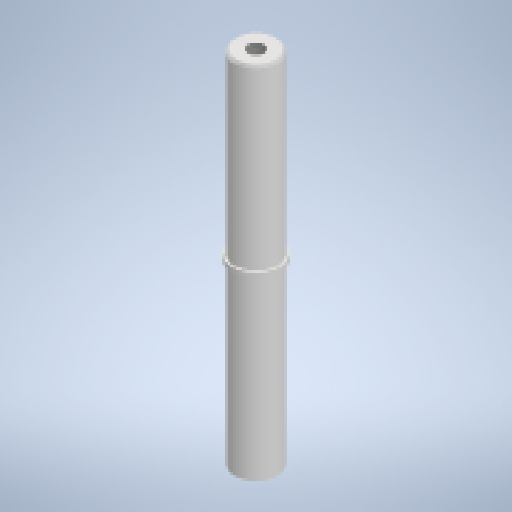
# Autodesk Inventor part: приводной вал
Saved by Autodesk Inventor 2024.2 (Build 282272000, 272)
## iProperties
Created: 2023-08-07
Part Number: приводной вал
Material: Generic
Document SubType Name: Modeling
Designer: admin
Density: 1 g/cm^3
Appearance: Default
Author: admin
Autodesk Inventor part; units mm, degrees
ref_plane "XZ Plane" through (0, 0, 0) normal (0, 1, 0) x (-1, 0, 0)
ref_plane "XY Plane" through (0, 0, 0) normal (0, 0, 1) x (1, 0, 0)
sketch "Sketch1" plane through (0, 0, 0) normal (0, 0, 1) x (1, 0, 0)
  line L0 (0, 75) -> (0, -75)
  line L1 (7, 75) -> (0, 75)
  line L2 (7, -75) -> (0, -75)
  line L3 (7, -75) -> (7, 75)
  line L4 (7, 1) -> (8, 1)
  line L5 (8, 1) -> (8, -1)
  line L6 (8, -1) -> (7, -1)
  point P0 (0, 0)
  point P1 (0, 0)
  point P2 (3.5, 75)
  point P3 (8, 0)
  dimension "d17" = 14
  dimension "d42" = 150
  dimension "d43" = 75
  dimension "d44" = 2
  dimension "d45" = 16
  constraints: 15 end point, 4 midpoint, 3 horizontal, 2 perpendicular, 2 point on line, 1 coincident, 1 vertical
  measures "d17" diameter of L3 L0
  measures "d42" distance of L2.start L1.start
  measures "d43" vertical distance of point (3.5, 75) point (8, 0)
  measures "d44" distance of L4.end L5.end
  measures "d45" diameter of L5 L0
revolve "Revolution1" add sketch "Sketch1" angle 360 about axis through (0, 75, 0) along (0, -1, 0)
sketch "Sketch4" plane through (0, 75, 0) normal (0, 1, 0) x (1, 0, 0)
  point P0 (0, 0)
  point P1 (0, 0)
  constraints: 1 coincident
hole "Hole1" at (0, 75, 0) direction (0, -1, 0) diameter 6.647 depth 22.2 tip angle 118 thread size "M8x1.25" class "6H" standard "ISO Metric profile"
chamfer "Chamfer1" distance 1 angle 45 1 edges at (-7, 75, 0)
ref_plane "Work Plane1" through (-7, -38, 0) normal (1, 0, 0) x (0, 1, 0)
sketch "Sketch5" plane through (-7, -38, 0) normal (1, 0, 0) x (0, 1, 0)
  line L0 (-37, 7) -> (-37, -7) projected
  line L1 (112, -7) -> (112, 7) projected
  line L2 (98, 0) -> (83, 0) construction
  line L3 (98, -2.5) -> (83, -2.5)
  line L4 (83, 2.5) -> (98, 2.5)
  arc A0 (98, -2.5) -> (98, 2.5) centre (98, 0) ccw
  arc A1 (83, 2.5) -> (83, -2.5) centre (83, 0) ccw
  line L5 (113, 6) -> (113, -6) projected
  line L6 (63, 0) -> (48, 0) construction
  line L7 (63, -2.5) -> (48, -2.5)
  line L8 (48, 2.5) -> (63, 2.5)
  arc A2 (63, -2.5) -> (63, 2.5) centre (63, 0) ccw
  arc A3 (48, 2.5) -> (48, -2.5) centre (48, 0) ccw
  point P0 (38, 0)
  point P1 (90.5, 0)
  point P2 (55.5, 0)
  dimension "d36" = 5
  dimension "d37" = 15
  dimension "d39" = 15
  dimension "d46" = 5
  dimension "d47" = 15
  dimension "d48" = 35
  constraints: 16 end point, 8 point on circle, 8 tangent, 4 centre point, 2 horizontal, 2 horizontal alignment, 2 midpoint, 2 parallel
  measures "d36" distance between parallel lines of L4 L3
  measures "d37" distance of L2.start L2.end
  measures "d39" distance from line of L2.start L5
  measures "d46" distance between parallel lines of L8 L7
  measures "d47" distance of L6.start L6.end
  measures "d48" distance of point (55.5, 0) point (90.5, 0)
extrude "Extrusion3" cut sketch "Sketch5" along normal blind 3
equation "\"d47\" = d37"
equation "\"d43\" = 0.5 * d42"
body "Solid1"
